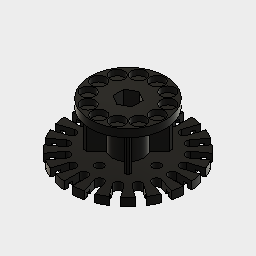
Wheel Back Plate (Autodesk Fusion 360 design; units mm, degrees)
Autodesk Fusion 360 part; units mm, degrees
sketch "Sketch1" plane through (0, 0, 0) normal (0, 1, 0) x (1, 0, 0)
  line L0 (0, 0) -> (0, -11)
  circle A0 centre (0, -11) radius 1.6
  line L1 (0, 0) -> (11, 0)
  circle A1 centre (11, 0) radius 1.6
  line L2 (0, 0) -> (-11, 0)
  circle A2 centre (-11, 0) radius 1.6
  line L3 (0, 0) -> (0, 11)
  circle A3 centre (0, 11) radius 1.6
  circle A4 centre (0, 0) radius 1.6
  line L4 (0, 0) -> (0, 22.5) construction
  line L5 (1.6, 22.443) -> (1.6, 17.1)
  line L6 (0, 15.5) -> (0, 15.5)
  line L7 (-1.6, 17.1) -> (-1.6, 22.443)
  arc A5 (-1.6, 17.1) -> (0, 15.5) centre (0, 17.1) ccw
  arc A6 (0, 15.5) -> (1.6, 17.1) centre (0, 17.1) ccw
  arc A7 (-4.7898, 14.7414) -> (-3.7625, 16.7575) centre (-5.2842, 16.2631) ccw
  arc A8 (-6.8059, 15.7686) -> (-4.7898, 14.7414) centre (-5.2842, 16.2631) ccw
  line L8 (-6.8059, 15.7686) -> (-8.457, 20.8502)
  line L9 (-5.4136, 21.839) -> (-3.7625, 16.7575)
  arc A9 (-9.1107, 12.5398) -> (-8.7567, 14.7746) centre (-10.0511, 13.8342) ccw
  arc A10 (-11.3456, 12.8937) -> (-9.1107, 12.5398) centre (-10.0511, 13.8342) ccw
  line L10 (-11.3456, 12.8937) -> (-14.4861, 17.2163)
  line L11 (-11.8973, 19.0973) -> (-8.7567, 14.7746)
  arc A11 (-12.5398, 9.1107) -> (-12.8937, 11.3456) centre (-13.8342, 10.0511) ccw
  arc A12 (-14.7746, 8.7567) -> (-12.5398, 9.1107) centre (-13.8342, 10.0511) ccw
  line L12 (-14.7746, 8.7567) -> (-19.0973, 11.8973)
  line L13 (-17.2163, 14.4861) -> (-12.8937, 11.3456)
  arc A13 (-14.7414, 4.7898) -> (-15.7686, 6.8059) centre (-16.2631, 5.2842) ccw
  arc A14 (-16.7575, 3.7625) -> (-14.7414, 4.7898) centre (-16.2631, 5.2842) ccw
  line L14 (-16.7575, 3.7625) -> (-21.839, 5.4136)
  line L15 (-20.8502, 8.457) -> (-15.7686, 6.8059)
  arc A15 (-15.5, 0) -> (-17.1, 1.6) centre (-17.1, 0) ccw
  arc A16 (-17.1, -1.6) -> (-15.5, 0) centre (-17.1, 0) ccw
  line L16 (-17.1, -1.6) -> (-22.443, -1.6)
  line L17 (-22.443, 1.6) -> (-17.1, 1.6)
  arc A17 (-14.7414, -4.7898) -> (-16.7575, -3.7625) centre (-16.2631, -5.2842) ccw
  arc A18 (-15.7686, -6.8059) -> (-14.7414, -4.7898) centre (-16.2631, -5.2842) ccw
  line L18 (-15.7686, -6.8059) -> (-20.8502, -8.457)
  line L19 (-21.839, -5.4136) -> (-16.7575, -3.7625)
  arc A19 (-12.5398, -9.1107) -> (-14.7746, -8.7567) centre (-13.8342, -10.0511) ccw
  arc A20 (-12.8937, -11.3456) -> (-12.5398, -9.1107) centre (-13.8342, -10.0511) ccw
  line L20 (-12.8937, -11.3456) -> (-17.2163, -14.4861)
  line L21 (-19.0973, -11.8973) -> (-14.7746, -8.7567)
  arc A21 (-9.1107, -12.5398) -> (-11.3456, -12.8937) centre (-10.0511, -13.8342) ccw
  arc A22 (-8.7567, -14.7746) -> (-9.1107, -12.5398) centre (-10.0511, -13.8342) ccw
  line L22 (-8.7567, -14.7746) -> (-11.8973, -19.0973)
  line L23 (-14.4861, -17.2163) -> (-11.3456, -12.8937)
  arc A23 (-4.7898, -14.7414) -> (-6.8059, -15.7686) centre (-5.2842, -16.2631) ccw
  arc A24 (-3.7625, -16.7575) -> (-4.7898, -14.7414) centre (-5.2842, -16.2631) ccw
  line L24 (-3.7625, -16.7575) -> (-5.4136, -21.839)
  line L25 (-8.457, -20.8502) -> (-6.8059, -15.7686)
  arc A25 (0, -15.5) -> (-1.6, -17.1) centre (0, -17.1) ccw
  arc A26 (1.6, -17.1) -> (0, -15.5) centre (0, -17.1) ccw
  line L26 (1.6, -17.1) -> (1.6, -22.443)
  line L27 (-1.6, -22.443) -> (-1.6, -17.1)
  arc A27 (4.7898, -14.7414) -> (3.7625, -16.7575) centre (5.2842, -16.2631) ccw
  arc A28 (6.8059, -15.7686) -> (4.7898, -14.7414) centre (5.2842, -16.2631) ccw
  line L28 (6.8059, -15.7686) -> (8.457, -20.8502)
  line L29 (5.4136, -21.839) -> (3.7625, -16.7575)
  arc A29 (9.1107, -12.5398) -> (8.7567, -14.7746) centre (10.0511, -13.8342) ccw
  arc A30 (11.3456, -12.8937) -> (9.1107, -12.5398) centre (10.0511, -13.8342) ccw
  line L30 (11.3456, -12.8937) -> (14.4861, -17.2163)
  line L31 (11.8973, -19.0973) -> (8.7567, -14.7746)
  arc A31 (12.5398, -9.1107) -> (12.8937, -11.3456) centre (13.8342, -10.0511) ccw
  arc A32 (14.7746, -8.7567) -> (12.5398, -9.1107) centre (13.8342, -10.0511) ccw
  line L32 (14.7746, -8.7567) -> (19.0973, -11.8973)
  line L33 (17.2163, -14.4861) -> (12.8937, -11.3456)
  arc A33 (14.7414, -4.7898) -> (15.7686, -6.8059) centre (16.2631, -5.2842) ccw
  arc A34 (16.7575, -3.7625) -> (14.7414, -4.7898) centre (16.2631, -5.2842) ccw
  line L34 (16.7575, -3.7625) -> (21.839, -5.4136)
  line L35 (20.8502, -8.457) -> (15.7686, -6.8059)
  arc A35 (15.5, 0) -> (17.1, -1.6) centre (17.1, 0) ccw
  arc A36 (17.1, 1.6) -> (15.5, 0) centre (17.1, 0) ccw
  line L36 (17.1, 1.6) -> (22.443, 1.6)
  line L37 (22.443, -1.6) -> (17.1, -1.6)
  arc A37 (14.7414, 4.7898) -> (16.7575, 3.7625) centre (16.2631, 5.2842) ccw
  arc A38 (15.7686, 6.8059) -> (14.7414, 4.7898) centre (16.2631, 5.2842) ccw
  line L38 (15.7686, 6.8059) -> (20.8502, 8.457)
  line L39 (21.839, 5.4136) -> (16.7575, 3.7625)
  arc A39 (12.5398, 9.1107) -> (14.7746, 8.7567) centre (13.8342, 10.0511) ccw
  arc A40 (12.8937, 11.3456) -> (12.5398, 9.1107) centre (13.8342, 10.0511) ccw
  line L40 (12.8937, 11.3456) -> (17.2163, 14.4861)
  line L41 (19.0973, 11.8973) -> (14.7746, 8.7567)
  arc A41 (9.1107, 12.5398) -> (11.3456, 12.8937) centre (10.0511, 13.8342) ccw
  arc A42 (8.7567, 14.7746) -> (9.1107, 12.5398) centre (10.0511, 13.8342) ccw
  line L42 (8.7567, 14.7746) -> (11.8973, 19.0973)
  line L43 (14.4861, 17.2163) -> (11.3456, 12.8937)
  arc A43 (4.7898, 14.7414) -> (6.8059, 15.7686) centre (5.2842, 16.2631) ccw
  arc A44 (3.7625, 16.7575) -> (4.7898, 14.7414) centre (5.2842, 16.2631) ccw
  line L44 (3.7625, 16.7575) -> (5.4136, 21.839)
  line L45 (8.457, 20.8502) -> (6.8059, 15.7686)
  line L46 (-1.6, -22.443) -> (-1.6, -22.9443)
  line L47 (1.6, -22.443) -> (1.6, -22.9443)
  line L48 (8.457, -20.8502) -> (8.6119, -21.3269)
  line L49 (5.4136, -21.839) -> (5.5685, -22.3157)
  line L50 (14.4861, -17.2163) -> (14.7807, -17.6219)
  line L51 (11.8973, -19.0973) -> (12.1919, -19.5028)
  line L52 (19.0973, -11.8973) -> (19.5028, -12.1919)
  line L53 (17.2163, -14.4861) -> (17.6219, -14.7807)
  line L54 (21.839, -5.4136) -> (22.3157, -5.5685)
  line L55 (20.8502, -8.457) -> (21.3269, -8.6119)
  line L56 (22.443, 1.6) -> (22.9443, 1.6)
  line L57 (22.443, -1.6) -> (22.9443, -1.6)
  line L58 (20.8502, 8.457) -> (21.3269, 8.6119)
  line L59 (21.839, 5.4136) -> (22.3157, 5.5685)
  line L60 (17.2163, 14.4861) -> (17.6219, 14.7807)
  line L61 (19.0973, 11.8973) -> (19.5028, 12.1919)
  line L62 (11.8973, 19.0973) -> (12.1919, 19.5028)
  line L63 (14.4861, 17.2163) -> (14.7807, 17.6219)
  line L64 (5.4136, 21.839) -> (5.5685, 22.3157)
  line L65 (8.457, 20.8502) -> (8.6119, 21.3269)
  line L66 (-1.6, 22.443) -> (-1.6, 22.9443)
  line L67 (1.6, 22.443) -> (1.6, 22.9443)
  line L68 (-8.457, 20.8502) -> (-8.6119, 21.3269)
  line L69 (-5.4136, 21.839) -> (-5.5685, 22.3157)
  line L70 (-14.4861, 17.2163) -> (-14.7807, 17.6219)
  line L71 (-11.8973, 19.0973) -> (-12.1919, 19.5028)
  line L72 (-19.0973, 11.8973) -> (-19.5028, 12.1919)
  line L73 (-17.2163, 14.4861) -> (-17.6219, 14.7807)
  line L74 (-21.839, 5.4136) -> (-22.3157, 5.5685)
  line L75 (-20.8502, 8.457) -> (-21.3269, 8.6119)
  line L76 (-22.443, -1.6) -> (-22.9443, -1.6)
  line L77 (-22.443, 1.6) -> (-22.9443, 1.6)
  line L78 (-20.8502, -8.457) -> (-21.3269, -8.6119)
  line L79 (-21.839, -5.4136) -> (-22.3157, -5.5685)
  line L80 (-17.2163, -14.4861) -> (-17.6219, -14.7807)
  line L81 (-19.0973, -11.8973) -> (-19.5028, -12.1919)
  line L82 (-11.8973, -19.0973) -> (-12.1919, -19.5028)
  line L83 (-14.4861, -17.2163) -> (-14.7807, -17.6219)
  line L84 (-5.4136, -21.839) -> (-5.5685, -22.3157)
  line L85 (-8.457, -20.8502) -> (-8.6119, -21.3269)
  arc A45 (17.6219, 14.7807) -> (14.7807, 17.6219) centre (0, 0) ccw
  arc A46 (12.1919, 19.5028) -> (8.6119, 21.3269) centre (0, 0) ccw
  arc A47 (5.5685, 22.3157) -> (1.6, 22.9443) centre (0, 0) ccw
  arc A48 (-1.6, 22.9443) -> (-5.5685, 22.3157) centre (0, 0) ccw
  arc A49 (-8.6119, 21.3269) -> (-12.1919, 19.5028) centre (0, 0) ccw
  arc A50 (-14.7807, 17.6219) -> (-17.6219, 14.7807) centre (0, 0) ccw
  arc A51 (-19.5028, 12.1919) -> (-21.3269, 8.6119) centre (0, 0) ccw
  arc A52 (-22.3157, 5.5685) -> (-22.9443, 1.6) centre (0, 0) ccw
  arc A53 (-22.9443, -1.6) -> (-22.3157, -5.5685) centre (0, 0) ccw
  arc A54 (-21.3269, -8.6119) -> (-19.5028, -12.1919) centre (0, 0) ccw
  arc A55 (-17.6219, -14.7807) -> (-14.7807, -17.6219) centre (0, 0) ccw
  arc A56 (-12.1919, -19.5028) -> (-8.6119, -21.3269) centre (0, 0) ccw
  arc A57 (-5.5685, -22.3157) -> (-1.6, -22.9443) centre (0, 0) ccw
  arc A58 (1.6, -22.9443) -> (5.5685, -22.3157) centre (0, 0) ccw
  arc A59 (8.6119, -21.3269) -> (12.1919, -19.5028) centre (0, 0) ccw
  arc A60 (14.7807, -17.6219) -> (17.6219, -14.7807) centre (0, 0) ccw
  arc A61 (19.5028, -12.1919) -> (21.3269, -8.6119) centre (0, 0) ccw
  arc A62 (22.3157, -5.5685) -> (22.9443, -1.6) centre (0, 0) ccw
  arc A63 (22.9443, 1.6) -> (22.3157, 5.5685) centre (0, 0) ccw
  arc A64 (21.3269, 8.6119) -> (19.5028, 12.1919) centre (0, 0) ccw
  point P0 (1.6, 15.5)
  point P1 (-1.6, 15.5)
  dimension "d10" = 3.2
  dimension "d11" = 11
  dimension "d12" = 3.2
  dimension "d13" = 11
  dimension "d14" = 3.2
  dimension "d15" = 11
  dimension "d16" = 3.2
  dimension "d17" = 3.2
  dimension "d51" = 3.2
  dimension "d53" = 1.6
  dimension "d55" = 360
  dimension "d59" = 46
  measures "d10" diameter of A0
  measures "d11" distance of L0.start L1.end
  measures "d12" diameter of A1
  measures "d13" distance of L0.start L2.end
  measures "d14" diameter of A2
  measures "d15" distance of L0.start L3.end
  measures "d16" diameter of A3
  measures "d17" diameter of A4
  measures "d51" distance of P0 P1
  measures "d53" radius of A5
  measures "d59" diameter of A45
extrude "Extrude1" add sketch "Sketch1" along normal blind 3
sketch "Sketch2" plane through (0, 0, 0) normal (0, -1, 0) x (1, 0, 0)
  circle A0 centre (0, -11) radius 1.6
  circle A1 centre (0, 11) radius 1.6
  circle A2 centre (-11, 0) radius 1.6
  circle A3 centre (11, 0) radius 1.6
  circle A4 centre (0, 0) radius 1.6
  circle A5 centre (0, 0) radius 19.9
  circle A6 centre (0, 0) radius 21.5
  line L0 (12.1919, -19.5028) -> (8.7567, -14.7746)
  arc A7 (11.3456, -12.8937) -> (8.7567, -14.7746) centre (10.0511, -13.8342) ccw
  line L1 (11.3456, -12.8937) -> (14.7807, -17.6219)
  line L2 (17.6219, -14.7807) -> (12.8937, -11.3456)
  arc A8 (14.7746, -8.7567) -> (12.8937, -11.3456) centre (13.8342, -10.0511) ccw
  line L3 (14.7746, -8.7567) -> (19.5028, -12.1919)
  line L4 (21.3269, -8.6119) -> (15.7686, -6.8059)
  arc A9 (16.7575, -3.7625) -> (15.7686, -6.8059) centre (16.2631, -5.2842) ccw
  line L5 (16.7575, -3.7625) -> (22.3157, -5.5685)
  line L6 (22.9443, -1.6) -> (17.1, -1.6)
  arc A10 (17.1, 1.6) -> (17.1, -1.6) centre (17.1, 0) ccw
  line L7 (17.1, 1.6) -> (22.9443, 1.6)
  line L8 (22.3157, 5.5685) -> (16.7575, 3.7625)
  arc A11 (15.7686, 6.8059) -> (16.7575, 3.7625) centre (16.2631, 5.2842) ccw
  line L9 (15.7686, 6.8059) -> (21.3269, 8.6119)
  line L10 (19.5028, 12.1919) -> (14.7746, 8.7567)
  arc A12 (12.8937, 11.3456) -> (14.7746, 8.7567) centre (13.8342, 10.0511) ccw
  line L11 (12.8937, 11.3456) -> (17.6219, 14.7807)
  line L12 (14.7807, 17.6219) -> (11.3456, 12.8937)
  arc A13 (8.7567, 14.7746) -> (11.3456, 12.8937) centre (10.0511, 13.8342) ccw
  line L13 (8.7567, 14.7746) -> (12.1919, 19.5028)
  line L14 (8.6119, 21.3269) -> (6.8059, 15.7686)
  arc A14 (3.7625, 16.7575) -> (6.8059, 15.7686) centre (5.2842, 16.2631) ccw
  line L15 (3.7625, 16.7575) -> (5.5685, 22.3157)
  line L16 (1.6, 22.9443) -> (1.6, 17.1)
  arc A15 (-1.6, 17.1) -> (1.6, 17.1) centre (0, 17.1) ccw
  line L17 (-1.6, 17.1) -> (-1.6, 22.9443)
  line L18 (-5.5685, 22.3157) -> (-3.7625, 16.7575)
  arc A16 (-6.8059, 15.7686) -> (-3.7625, 16.7575) centre (-5.2842, 16.2631) ccw
  line L19 (-6.8059, 15.7686) -> (-8.6119, 21.3269)
  line L20 (-12.1919, 19.5028) -> (-8.7567, 14.7746)
  arc A17 (-11.3456, 12.8937) -> (-8.7567, 14.7746) centre (-10.0511, 13.8342) ccw
  line L21 (-11.3456, 12.8937) -> (-14.7807, 17.6219)
  line L22 (-17.6219, 14.7807) -> (-12.8937, 11.3456)
  arc A18 (-14.7746, 8.7567) -> (-12.8937, 11.3456) centre (-13.8342, 10.0511) ccw
  line L23 (-14.7746, 8.7567) -> (-19.5028, 12.1919)
  line L24 (-21.3269, 8.6119) -> (-15.7686, 6.8059)
  arc A19 (-16.7575, 3.7625) -> (-15.7686, 6.8059) centre (-16.2631, 5.2842) ccw
  line L25 (-16.7575, 3.7625) -> (-22.3157, 5.5685)
  line L26 (-22.9443, 1.6) -> (-17.1, 1.6)
  arc A20 (-17.1, -1.6) -> (-17.1, 1.6) centre (-17.1, 0) ccw
  line L27 (-17.1, -1.6) -> (-22.9443, -1.6)
  line L28 (-22.3157, -5.5685) -> (-16.7575, -3.7625)
  arc A21 (-15.7686, -6.8059) -> (-16.7575, -3.7625) centre (-16.2631, -5.2842) ccw
  line L29 (-15.7686, -6.8059) -> (-21.3269, -8.6119)
  line L30 (-19.5028, -12.1919) -> (-14.7746, -8.7567)
  arc A22 (-12.8937, -11.3456) -> (-14.7746, -8.7567) centre (-13.8342, -10.0511) ccw
  line L31 (-12.8937, -11.3456) -> (-17.6219, -14.7807)
  line L32 (-14.7807, -17.6219) -> (-11.3456, -12.8937)
  arc A23 (-8.7567, -14.7746) -> (-11.3456, -12.8937) centre (-10.0511, -13.8342) ccw
  line L33 (-8.7567, -14.7746) -> (-12.1919, -19.5028)
  line L34 (-8.6119, -21.3269) -> (-6.8059, -15.7686)
  arc A24 (-3.7625, -16.7575) -> (-6.8059, -15.7686) centre (-5.2842, -16.2631) ccw
  line L35 (-3.7625, -16.7575) -> (-5.5685, -22.3157)
  line L36 (-1.6, -22.9443) -> (-1.6, -17.1)
  arc A25 (1.6, -17.1) -> (-1.6, -17.1) centre (0, -17.1) ccw
  line L37 (1.6, -17.1) -> (1.6, -22.9443)
  line L38 (5.5685, -22.3157) -> (3.7625, -16.7575)
  arc A26 (6.8059, -15.7686) -> (3.7625, -16.7575) centre (5.2842, -16.2631) ccw
  line L39 (6.8059, -15.7686) -> (8.6119, -21.3269)
  arc A27 (22.3157, -5.5685) -> (22.9443, -1.6) centre (0, 0) ccw
  arc A28 (22.9443, 1.6) -> (22.3157, 5.5685) centre (0, 0) ccw
  arc A29 (21.3269, 8.6119) -> (19.5028, 12.1919) centre (0, 0) ccw
  arc A30 (17.6219, 14.7807) -> (14.7807, 17.6219) centre (0, 0) ccw
  arc A31 (12.1919, 19.5028) -> (8.6119, 21.3269) centre (0, 0) ccw
  arc A32 (5.5685, 22.3157) -> (1.6, 22.9443) centre (0, 0) ccw
  arc A33 (-1.6, 22.9443) -> (-5.5685, 22.3157) centre (0, 0) ccw
  arc A34 (-8.6119, 21.3269) -> (-12.1919, 19.5028) centre (0, 0) ccw
  arc A35 (-14.7807, 17.6219) -> (-17.6219, 14.7807) centre (0, 0) ccw
  arc A36 (-19.5028, 12.1919) -> (-21.3269, 8.6119) centre (0, 0) ccw
  arc A37 (-22.3157, 5.5685) -> (-22.9443, 1.6) centre (0, 0) ccw
  arc A38 (-22.9443, -1.6) -> (-22.3157, -5.5685) centre (0, 0) ccw
  arc A39 (-21.3269, -8.6119) -> (-19.5028, -12.1919) centre (0, 0) ccw
  arc A40 (-17.6219, -14.7807) -> (-14.7807, -17.6219) centre (0, 0) ccw
  arc A41 (-12.1919, -19.5028) -> (-8.6119, -21.3269) centre (0, 0) ccw
  arc A42 (-5.5685, -22.3157) -> (-1.6, -22.9443) centre (0, 0) ccw
  arc A43 (1.6, -22.9443) -> (5.5685, -22.3157) centre (0, 0) ccw
  arc A44 (8.6119, -21.3269) -> (12.1919, -19.5028) centre (0, 0) ccw
  arc A45 (14.7807, -17.6219) -> (17.6219, -14.7807) centre (0, 0) ccw
  arc A46 (19.5028, -12.1919) -> (21.3269, -8.6119) centre (0, 0) ccw
  dimension "d20" = 39.8
  dimension "d21" = 43
  measures "d20" diameter of A5
  measures "d21" diameter of A6
extrude "Extrude2" cut sketch "Sketch2" against normal blind 1.4 contours A5 A6 L6 L7 | A5 A6 L7 L8 | A5 A6 L5 L6 | A5 A6 L8 L9 | A5 A6 L4 L5 | A5 A6 L9 L10 | A5 A6 L3 L4 | A5 A6 L10 L11 | A5 A6 L2 L3 | A5 A6 L11 L12 | A5 A6 L1 L2 | A5 A6 L12 L13 | A5 A6 L0 L1 | A5 A6 L13 L14 | A5 A6 L0 L39 | A5 A6 L14 L15 | A5 A6 L38 L39 | A5 A6 L15 L16 | A5 A6 L37 L38 | A5 A6 L16 L17 | A5 A6 L36 L37 | A5 A6 L17 L18 | A5 A6 L35 L36 | A5 A6 L18 L19 | A5 A6 L34 L35 | A5 A6 L19 L20 | A5 A6 L33 L34 | A5 A6 L20 L21 | A5 A6 L32 L33 | A5 A6 L21 L22 | A5 A6 L31 L32 | A5 A6 L22 L23 | A5 A6 L30 L31 | A5 A6 L23 L24 | A5 A6 L29 L30 | A5 A6 L24 L25 | A5 A6 L28 L29 | A5 A6 L25 L26 | A5 A6 L27 L28 | A5 A6 L26 L27
sketch "Sketch3" plane through (0, 3, 0) normal (0, 1, 0) x (-1, 0, 0)
  circle A0 centre (0, -11) radius 1.6
  circle A1 centre (0, 11) radius 1.6
  circle A2 centre (11, 0) radius 1.6
  circle A3 centre (-11, 0) radius 1.6
  circle A4 centre (0, 0) radius 1.6
  circle A5 centre (0, 0) radius 6
  line L0 (-3.7, -2.1362) -> (0, -4.2724)
  line L1 (0, -4.2724) -> (3.7, -2.1362)
  line L2 (3.7, -2.1362) -> (3.7, 2.1362)
  line L3 (3.7, 2.1362) -> (0, 4.2724)
  line L4 (0, 4.2724) -> (-3.7, 2.1362)
  line L5 (-3.7, 2.1362) -> (-3.7, -2.1362)
  line L6 (0, 0) -> (10, 0) construction
  line L7 (0.7071, 0.7071) -> (-7.7782, 9.1924)
  line L8 (-0.7071, -0.7071) -> (-9.1924, 7.7782)
  line L9 (-7.7782, 9.1924) -> (-9.1924, 7.7782)
  line L10 (0.7071, -0.7071) -> (-7.7782, -9.1924)
  line L11 (-9.1924, -7.7782) -> (-7.7782, -9.1924)
  line L12 (-0.7071, 0.7071) -> (-9.1924, -7.7782)
  line L13 (0.7071, 0.7071) -> (9.1924, -7.7782)
  line L14 (7.7782, -9.1924) -> (9.1924, -7.7782)
  line L15 (-0.7071, -0.7071) -> (7.7782, -9.1924)
  line L16 (-0.7071, 0.7071) -> (7.7782, 9.1924)
  line L17 (9.1924, 7.7782) -> (7.7782, 9.1924)
  line L18 (0.7071, -0.7071) -> (9.1924, 7.7782)
  line L19 (-8.7567, -14.7746) -> (-12.1919, -19.5028)
  line L20 (-8.6119, -21.3269) -> (-6.8059, -15.7686)
  arc A6 (-3.7625, -16.7575) -> (-6.8059, -15.7686) centre (-5.2842, -16.2631) ccw
  line L21 (-3.7625, -16.7575) -> (-5.5685, -22.3157)
  line L22 (-1.6, -22.9443) -> (-1.6, -17.1)
  arc A7 (1.6, -17.1) -> (-1.6, -17.1) centre (0, -17.1) ccw
  line L23 (1.6, -17.1) -> (1.6, -22.9443)
  line L24 (5.5685, -22.3157) -> (3.7625, -16.7575)
  arc A8 (6.8059, -15.7686) -> (3.7625, -16.7575) centre (5.2842, -16.2631) ccw
  line L25 (6.8059, -15.7686) -> (8.6119, -21.3269)
  line L26 (12.1919, -19.5028) -> (8.7567, -14.7746)
  arc A9 (11.3456, -12.8937) -> (8.7567, -14.7746) centre (10.0511, -13.8342) ccw
  line L27 (11.3456, -12.8937) -> (14.7807, -17.6219)
  line L28 (17.6219, -14.7807) -> (12.8937, -11.3456)
  arc A10 (14.7746, -8.7567) -> (12.8937, -11.3456) centre (13.8342, -10.0511) ccw
  line L29 (14.7746, -8.7567) -> (19.5028, -12.1919)
  line L30 (21.3269, -8.6119) -> (15.7686, -6.8059)
  arc A11 (16.7575, -3.7625) -> (15.7686, -6.8059) centre (16.2631, -5.2842) ccw
  line L31 (16.7575, -3.7625) -> (22.3157, -5.5685)
  line L32 (22.9443, -1.6) -> (17.1, -1.6)
  arc A12 (17.1, 1.6) -> (17.1, -1.6) centre (17.1, 0) ccw
  line L33 (17.1, 1.6) -> (22.9443, 1.6)
  line L34 (22.3157, 5.5685) -> (16.7575, 3.7625)
  arc A13 (15.7686, 6.8059) -> (16.7575, 3.7625) centre (16.2631, 5.2842) ccw
  line L35 (15.7686, 6.8059) -> (21.3269, 8.6119)
  line L36 (19.5028, 12.1919) -> (14.7746, 8.7567)
  arc A14 (12.8937, 11.3456) -> (14.7746, 8.7567) centre (13.8342, 10.0511) ccw
  line L37 (12.8937, 11.3456) -> (17.6219, 14.7807)
  line L38 (14.7807, 17.6219) -> (11.3456, 12.8937)
  arc A15 (8.7567, 14.7746) -> (11.3456, 12.8937) centre (10.0511, 13.8342) ccw
  line L39 (8.7567, 14.7746) -> (12.1919, 19.5028)
  line L40 (8.6119, 21.3269) -> (6.8059, 15.7686)
  arc A16 (3.7625, 16.7575) -> (6.8059, 15.7686) centre (5.2842, 16.2631) ccw
  line L41 (3.7625, 16.7575) -> (5.5685, 22.3157)
  line L42 (1.6, 22.9443) -> (1.6, 17.1)
  arc A17 (-1.6, 17.1) -> (1.6, 17.1) centre (0, 17.1) ccw
  line L43 (-1.6, 17.1) -> (-1.6, 22.9443)
  line L44 (-5.5685, 22.3157) -> (-3.7625, 16.7575)
  arc A18 (-6.8059, 15.7686) -> (-3.7625, 16.7575) centre (-5.2842, 16.2631) ccw
  line L45 (-6.8059, 15.7686) -> (-8.6119, 21.3269)
  line L46 (-12.1919, 19.5028) -> (-8.7567, 14.7746)
  arc A19 (-11.3456, 12.8937) -> (-8.7567, 14.7746) centre (-10.0511, 13.8342) ccw
  line L47 (-11.3456, 12.8937) -> (-14.7807, 17.6219)
  line L48 (-17.6219, 14.7807) -> (-12.8937, 11.3456)
  arc A20 (-14.7746, 8.7567) -> (-12.8937, 11.3456) centre (-13.8342, 10.0511) ccw
  line L49 (-14.7746, 8.7567) -> (-19.5028, 12.1919)
  line L50 (-21.3269, 8.6119) -> (-15.7686, 6.8059)
  arc A21 (-16.7575, 3.7625) -> (-15.7686, 6.8059) centre (-16.2631, 5.2842) ccw
  line L51 (-16.7575, 3.7625) -> (-22.3157, 5.5685)
  line L52 (-22.9443, 1.6) -> (-17.1, 1.6)
  arc A22 (-17.1, -1.6) -> (-17.1, 1.6) centre (-17.1, 0) ccw
  line L53 (-17.1, -1.6) -> (-22.9443, -1.6)
  line L54 (-22.3157, -5.5685) -> (-16.7575, -3.7625)
  arc A23 (-15.7686, -6.8059) -> (-16.7575, -3.7625) centre (-16.2631, -5.2842) ccw
  line L55 (-15.7686, -6.8059) -> (-21.3269, -8.6119)
  line L56 (-19.5028, -12.1919) -> (-14.7746, -8.7567)
  arc A24 (-12.8937, -11.3456) -> (-14.7746, -8.7567) centre (-13.8342, -10.0511) ccw
  line L57 (-12.8937, -11.3456) -> (-17.6219, -14.7807)
  line L58 (-14.7807, -17.6219) -> (-11.3456, -12.8937)
  arc A25 (-8.7567, -14.7746) -> (-11.3456, -12.8937) centre (-10.0511, -13.8342) ccw
  arc A26 (-21.3269, -8.6119) -> (-19.5028, -12.1919) centre (0, 0) ccw
  arc A27 (-17.6219, -14.7807) -> (-14.7807, -17.6219) centre (0, 0) ccw
  arc A28 (-12.1919, -19.5028) -> (-8.6119, -21.3269) centre (0, 0) ccw
  arc A29 (-5.5685, -22.3157) -> (-1.6, -22.9443) centre (0, 0) ccw
  arc A30 (1.6, -22.9443) -> (5.5685, -22.3157) centre (0, 0) ccw
  arc A31 (8.6119, -21.3269) -> (12.1919, -19.5028) centre (0, 0) ccw
  arc A32 (14.7807, -17.6219) -> (17.6219, -14.7807) centre (0, 0) ccw
  arc A33 (19.5028, -12.1919) -> (21.3269, -8.6119) centre (0, 0) ccw
  arc A34 (22.3157, -5.5685) -> (22.9443, -1.6) centre (0, 0) ccw
  arc A35 (22.9443, 1.6) -> (22.3157, 5.5685) centre (0, 0) ccw
  arc A36 (21.3269, 8.6119) -> (19.5028, 12.1919) centre (0, 0) ccw
  arc A37 (17.6219, 14.7807) -> (14.7807, 17.6219) centre (0, 0) ccw
  arc A38 (12.1919, 19.5028) -> (8.6119, 21.3269) centre (0, 0) ccw
  arc A39 (5.5685, 22.3157) -> (1.6, 22.9443) centre (0, 0) ccw
  arc A40 (-1.6, 22.9443) -> (-5.5685, 22.3157) centre (0, 0) ccw
  arc A41 (-8.6119, 21.3269) -> (-12.1919, 19.5028) centre (0, 0) ccw
  arc A42 (-14.7807, 17.6219) -> (-17.6219, 14.7807) centre (0, 0) ccw
  arc A43 (-19.5028, 12.1919) -> (-21.3269, 8.6119) centre (0, 0) ccw
  arc A44 (-22.3157, 5.5685) -> (-22.9443, 1.6) centre (0, 0) ccw
  arc A45 (-22.9443, -1.6) -> (-22.3157, -5.5685) centre (0, 0) ccw
  dimension "d25" = 12
  dimension "d28" = 3.7
  dimension "d46" = 360
  measures "d25" diameter of A5
  measures "d28" distance of A4.centre L5
extrude "Extrude3" add sketch "Sketch3" along normal blind 14 contours A5 L1 L2 L3 L13 L18 | A5 L3 L16 L18 | A5 L1 L13 L15 | A5 L3 L4 L7 L16 | A5 L16 L17 L18 | A5 L0 L1 L10 L15 | A5 L13 L14 L15 | A5 L4 L7 L8 | A5 L0 L10 L12 | A5 L0 L4 L5 L8 L12 | A5 L7 L8 L9 | A5 L10 L11 L12
extrude "Extrude4" add 1 faces at (-1.5, 3, 2.5981) along direction (0, 1, 0) blind 6
sketch "Sketch4" plane through (0, 17, 0) normal (0, 1, 0) x (-1, 0, 0)
  line L0 (-3.7, -2.1362) -> (-3.7, 2.1362)
  line L1 (-3.7, 2.1362) -> (0, 4.2724)
  line L2 (0, 4.2724) -> (3.7, 2.1362)
  line L3 (3.7, 2.1362) -> (3.7, -2.1362)
  line L4 (3.7, -2.1362) -> (0, -4.2724)
  line L5 (0, -4.2724) -> (-3.7, -2.1362)
  circle A0 centre (0, 0) radius 14.5
  arc A1 (4.8904, -3.4762) -> (4.8904, 3.4762) centre (0, 0) ccw
  line L6 (4.8904, 3.4762) -> (9.1924, 7.7782)
  line L7 (9.1924, 7.7782) -> (7.7782, 9.1924)
  line L8 (7.7782, 9.1924) -> (3.4762, 4.8904)
  arc A2 (3.4762, 4.8904) -> (-3.4762, 4.8904) centre (0, 0) ccw
  line L9 (-3.4762, 4.8904) -> (-7.7782, 9.1924)
  line L10 (-7.7782, 9.1924) -> (-9.1924, 7.7782)
  line L11 (-9.1924, 7.7782) -> (-4.8904, 3.4762)
  arc A3 (-4.8904, 3.4762) -> (-4.8904, -3.4762) centre (0, 0) ccw
  line L12 (-4.8904, -3.4762) -> (-9.1924, -7.7782)
  line L13 (-9.1924, -7.7782) -> (-7.7782, -9.1924)
  line L14 (-7.7782, -9.1924) -> (-3.4762, -4.8904)
  arc A4 (-3.4762, -4.8904) -> (3.4762, -4.8904) centre (0, 0) ccw
  line L15 (3.4762, -4.8904) -> (7.7782, -9.1924)
  line L16 (7.7782, -9.1924) -> (9.1924, -7.7782)
  line L17 (9.1924, -7.7782) -> (4.8904, -3.4762)
  dimension "d31" = 29
  measures "d31" diameter of A0
extrude "Extrude5" add sketch "Sketch4" along normal blind 3 contours A0 | A1 L6 L7 L8 A2 L9 L10 L11 A3 L12 L13 L14 A4 L15 L16 L17
sketch "Sketch5" plane through (0, 20, 0) normal (0, 1, 0) x (-1, 0, 0)
  circle A0 centre (0, 0) radius 14.5
  circle A1 centre (-5.5994, -9.7575) radius 2.75
  circle A2 centre (9.7575, -5.5994) radius 2.75
  circle A3 centre (-9.728, -5.6505) radius 2.75
  circle A4 centre (11.2499, 0.0295) radius 2.75
  circle A5 centre (9.728, 5.6505) radius 2.75
  circle A6 centre (5.5994, 9.7575) radius 2.75
  circle A7 centre (-0.0295, 11.2499) radius 2.75
  circle A8 centre (-5.6505, 9.728) radius 2.75
  line L0 (0.0295, -7.9999) -> (0.0295, -11.2499)
  circle A9 centre (-9.7575, 5.5994) radius 2.75
  circle A10 centre (-11.2499, -0.0295) radius 2.75
  circle A11 centre (0, 0) radius 14.5
  circle A12 centre (5.6505, -9.728) radius 2.75
  circle A13 centre (0.0295, -11.2499) radius 2.75
  dimension "d37" = 3.25
  dimension "d38" = 5.5
  measures "d37" distance of L0.start L0.end
  measures "d38" diameter of A13
extrude "Extrude6" cut sketch "Sketch5" against normal blind 2.2 contours A1 | A2 | A3 | A4 | A5 | A6 | A7 | A8 | A9 | A10 | A12 | A13
chamfer "Chamfer2" distance 0.7 angle 45 8 edges at (7.7782, 10, 9.1924) (9.1924, 10, 7.7782) (9.1924, 10, -7.7782) (7.7782, 10, -9.1924) (-7.7782, 10, -9.1924) (-9.1924, 10, -7.7782) (-9.1924, 10, 7.7782) (-7.7782, 10, 9.1924)
